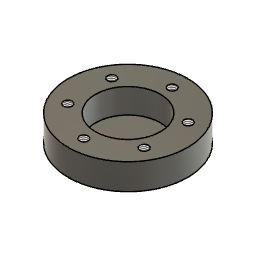
contact part v2 (Autodesk Fusion 360 design; units mm, degrees)
Autodesk Fusion 360 part; units mm, degrees
note: some values were not read from the file. Set by a fixed rule: the direction of a hole.
sketch "Sketch1" plane through (0, 0, 0) normal (0, 1, 0) x (1, 0, 0)
  circle A0 centre (0, 0) radius 23
  line L0 (-10, -15) -> (10, -15)
  line L1 (10, -15) -> (10, 15)
  line L2 (10, 15) -> (-10, 15)
  line L3 (-10, 15) -> (-10, -15)
  line L4 (1.75, 0) -> (22.5, 0) construction
  line L5 (0, -1.75) -> (0, -22.5) construction
  line L6 (-8, -14.25) -> (-12, -14.25)
  arc A1 (-12, -14.25) -> (-12, -15.75) centre (-12, -15) ccw
  line L7 (-12, -15.75) -> (-8, -15.75)
  arc A2 (-8, -15.75) -> (-8, -14.25) centre (-8, -15) ccw
  line L8 (-8, -15) -> (-12, -15) construction
  point P0 (-10, -15)
  point P1 (10, -15)
  point P2 (10, 15)
  point P3 (-10, 15)
  point P4 (-10, -15)
  point P5 (0, -17)
  dimension "d1" = 46
  dimension "d8" = 20
  dimension "d9" = 30
  dimension "d10" = 4
  dimension "d11" = 1.5
  dimension "d21" = 17
  constraint coincident A0.centre origin
  constraint horizontal L0
  constraint vertical L1
  constraint horizontal L2
  constraint vertical L3
  constraint symmetric L1 L3 L5
  constraint symmetric L0 L2 L4
  constraint coincident P4 P0
  constraint coincident P1 L0.end
  constraint coincident P2 L1.end
  constraint coincident P3 L2.end
  constraint tangent L6 A1
  constraint tangent A1 L7
  constraint parallel L6 L7
  constraint tangent L7 A2
  constraint tangent L6 A2
  constraint perpendicular L3 L8
  constraint midpoint L8 P4
  constraint coincident L5 P5
  measures "d1" diameter of A0
  measures "d8" distance of L1 L3
  measures "d9" distance of P1 P2
  measures "d10" distance of A2.centre A1.centre
  measures "d11" distance of L6 L7
  measures "d21" distance of A0.centre P5
extrude "Extrude1" add sketch "Sketch1" along normal blind 10 contours A0 | L0 L3 L6 A2 | L0 L3 L6 A1 L7 A2 | L0 L1 L2 L3 L6 A2
hole "Hole1" at (0, 10, 0) direction (0, -1, 0) diameter 25 depth 9.5 tip angle 180
hole "Hole2" at (-10, 0, 15) direction (0, 1, 0) diameter 3.332 depth 5 tip angle 180
thread "Thread2" "ISO Metric profile 4.0 M4x0.7 6H" thread offset 0 thread depth 10
extrude "Extrude2" cut sketch "Sketch1" along normal blind 4 contours L0 L3 L6 A2 | L0 L3 L6 A1 L7 A2
pattern_linear "R-Pattern1" count 2 spacing 20 along (1, 0, 0) count 2 spacing 30 along (0, 0, -1) of "Hole2", "Extrude2"
sketch "Sketch2" plane through (0, 10, 0) normal (0, 1, 0) x (-1, 0, 0)
  circle A0 centre (0, 0) radius 12.5
  circle A1 centre (0, 0) radius 23
  point P0 (0, 17)
hole "Hole3" at (0, 10, 17) direction (0, -1, 0) diameter 3.332 depth 5 tip angle 180
thread "Thread3" "ISO Metric profile 4.0 M4x0.7 6H" thread offset 0 thread depth 10
pattern_circular "C-Pattern1" count 6 over 360 about axis through (0, 1.75, 0) along (0, 1, 0) of "Hole3"
